Autodesk Fusion 360 part; units mm, degrees
(part 2 of 2)
sketch "Left" plane through (-18.285, 0, 0) normal (-1, 0, 0) x (0, 0, 1) in component "DXF Export"
  line L0 (-12.85, 17) -> (-12.85, 13)
  line L1 (-12.85, 13) -> (-17.35, 13)
  line L2 (-17.35, 13) -> (-17.35, 17)
  line L3 (-17.35, 17) -> (-12.85, 17)
  line L4 (23, -4) -> (23, 0)
  line L5 (23, 0) -> (27.5, 0)
  line L6 (27.5, 0) -> (27.5, 4.5)
  line L7 (27.5, 4.5) -> (31.5, 4.5)
  line L8 (31.5, 4.5) -> (31.5, 9)
  line L9 (31.5, 9) -> (27.5, 9)
  line L10 (27.5, 9) -> (27.5, 13.95)
  line L11 (27.5, 13.95) -> (26.8, 13.95)
  line L12 (26.8, 13.95) -> (26.8, 13.15)
  line L13 (26.8, 13.15) -> (25.4, 13.15)
  line L14 (25.4, 13.15) -> (25.4, 16.35)
  line L15 (25.4, 16.35) -> (26.8, 16.35)
  line L16 (26.8, 16.35) -> (26.8, 15.55)
  line L17 (26.8, 15.55) -> (27.5, 15.55)
  line L18 (27.5, 15.55) -> (27.5, 20.5)
  line L19 (27.5, 29.5) -> (23, 29.5)
  line L20 (23, 29.5) -> (23, 33.5)
  line L21 (23, 33.5) -> (18.5, 33.5)
  line L22 (18.5, 33.5) -> (18.5, 29.5)
  line L23 (18.5, 29.5) -> (0.8, 29.5)
  line L24 (0.8, 29.5) -> (0.8, 28.8)
  line L25 (0.8, 28.8) -> (1.6, 28.8)
  line L26 (1.6, 28.8) -> (1.6, 27.4)
  line L27 (1.6, 27.4) -> (-1.6, 27.4)
  line L28 (-1.6, 27.4) -> (-1.6, 28.8)
  line L29 (-1.6, 28.8) -> (-0.8, 28.8)
  line L30 (-0.8, 28.8) -> (-0.8, 29.5)
  line L31 (-0.8, 29.5) -> (-18.5, 29.5)
  line L32 (-18.5, 29.5) -> (-18.5, 33.5)
  line L33 (-18.5, 33.5) -> (-23, 33.5)
  line L34 (-23, 33.5) -> (-23, 29.5)
  line L35 (-23, 29.5) -> (-27.5, 29.5)
  line L36 (-27.5, 29.5) -> (-27.5, 25)
  line L37 (-27.5, 15.55) -> (-26.8, 15.55)
  line L38 (-26.8, 15.55) -> (-26.8, 16.35)
  line L39 (-26.8, 16.35) -> (-25.4, 16.35)
  line L40 (-25.4, 16.35) -> (-25.4, 13.15)
  line L41 (-25.4, 13.15) -> (-26.8, 13.15)
  line L42 (-26.8, 13.15) -> (-26.8, 13.95)
  line L43 (-26.8, 13.95) -> (-27.5, 13.95)
  line L44 (-27.5, 13.95) -> (-27.5, 9)
  line L45 (-27.5, 9) -> (-31.5, 9)
  line L46 (-31.5, 9) -> (-31.5, 4.5)
  line L47 (-31.5, 4.5) -> (-27.5, 4.5)
  line L48 (-27.5, 4.5) -> (-27.5, 0)
  line L49 (-27.5, 0) -> (-23, 0)
  line L50 (-23, 0) -> (-23, -4)
  line L51 (-23, -4) -> (-18.5, -4)
  line L52 (-18.5, -4) -> (-18.5, 0)
  line L53 (-18.5, 0) -> (-0.8, 0)
  line L54 (-0.8, 0) -> (-0.8, 0.7)
  line L55 (-0.8, 0.7) -> (-1.6, 0.7)
  line L56 (-1.6, 0.7) -> (-1.6, 2.1)
  line L57 (-1.6, 2.1) -> (1.6, 2.1)
  line L58 (1.6, 2.1) -> (1.6, 0.7)
  line L59 (1.6, 0.7) -> (0.8, 0.7)
  line L60 (0.8, 0.7) -> (0.8, 0)
  line L61 (0.8, 0) -> (18.5, 0)
  line L62 (18.5, 0) -> (18.5, -4)
  line L63 (18.5, -4) -> (23, -4)
  line L64 (27.5, 20.5) -> (31.5, 20.5)
  line L65 (31.5, 20.5) -> (31.5, 25)
  line L66 (31.5, 25) -> (27.5, 25)
  line L67 (27.5, 25) -> (27.5, 29.5)
  line L68 (-27.5, 25) -> (-31.5, 25)
  line L69 (-31.5, 25) -> (-31.5, 20.5)
  line L70 (-31.5, 20.5) -> (-27.5, 20.5)
  line L71 (-27.5, 20.5) -> (-27.5, 15.55)
sketch "Mid Plane" plane through (0, 17, 0) normal (0, 1, 0) x (-1, 0, 0) in component "DXF Export"
  line L0 (14.285, 27.5) -> (12.35, 27.5)
  line L1 (12.35, 27.5) -> (12.35, 31.5)
  line L2 (12.35, 31.5) -> (7.85, 31.5)
  line L3 (7.85, 31.5) -> (7.85, 27.5)
  line L4 (7.85, 27.5) -> (-14.285, 27.5)
  line L5 (-14.285, 27.5) -> (-14.285, 17.35)
  line L6 (-14.285, 17.35) -> (-18.285, 17.35)
  line L7 (-18.285, 17.35) -> (-18.285, 12.85)
  line L8 (-18.285, 12.85) -> (-14.285, 12.85)
  line L9 (-14.285, 12.85) -> (-14.285, -27.5)
  line L10 (-14.285, -27.5) -> (-12.35, -27.5)
  line L11 (-12.35, -27.5) -> (-12.35, -31.5)
  line L12 (-12.35, -31.5) -> (-7.85, -31.5)
  line L13 (-7.85, -31.5) -> (-7.85, -27.5)
  line L14 (-7.85, -27.5) -> (14.285, -27.5)
  line L15 (14.285, -27.5) -> (14.285, -17.35)
  line L16 (14.285, -17.35) -> (18.285, -17.35)
  line L17 (18.285, -17.35) -> (18.285, -12.85)
  line L18 (18.285, -12.85) -> (14.285, -12.85)
  line L19 (14.285, -12.85) -> (14.285, 27.5)
  line L20 (3.91, 10.1297) -> (-3.89, 10.1297)
  line L21 (-3.89, 10.1297) -> (-3.89, 24.1297)
  line L22 (-3.89, 24.1297) -> (3.91, 24.1297)
  line L23 (3.91, 24.1297) -> (3.91, 10.1297)
  line L24 (-10.165, 24.32) -> (-10.165, -24.52)
  line L25 (-10.165, -24.52) -> (-12.785, -24.52)
  line L26 (-12.785, -24.52) -> (-12.785, 24.32)
  line L27 (-12.785, 24.32) -> (-10.165, 24.32)
  line L28 (10.165, 24.32) -> (12.785, 24.32)
  line L29 (12.785, 24.32) -> (12.785, -24.52)
  line L30 (12.785, -24.52) -> (10.165, -24.52)
  line L31 (10.165, -24.52) -> (10.165, 24.32)
equation "d1 = object_length"
equation "d2 = object_width"
equation "d3 = tolerance_to_object"
equation "d4 = material_thickness + tolerance_to_object"
equation "d19 = object_height + tolerance_to_object * 2"
equation "d161 = 68.40 mm / 6"
equation "d199 = 4 mm"
equation "d210 = d199"
equation "d232 = d199"
equation "object_height = 26.5 mm"
equation "object_width = 25.57 mm"
equation "object_length = 52 mm"
equation "tolerance_to_object = 1.5 mm"
equation "pin_thickness = 4.5 mm"
equation "material_thickness = 4 mm"
equation "nut_width = 3.2 mm"
equation "nut_height = 1.4 mm"
equation "screw_length = 6.1 mm"
equation "screw_hole_diameter = 1.6 mm"
equation "d358 = object_height + 2 * tolerance_to_object"
equation "d361 = object_length / 2 + tolerance_to_object"
equation "d368 = d19 - pin_thickness"
equation "d385 = pin_thickness"
equation "d386 = pin_thickness"
equation "d387 = d386"
equation "d388 = pin_thickness"
equation "d389 = d388"
equation "d391 = pin_thickness"
equation "d392 = pin_thickness"
equation "d394 = d395"
equation "d395 = pin_thickness"
equation "d396 = d397"
equation "d397 = pin_thickness"
equation "d399 = pin_thickness"
equation "d401 = -d361"
equation "d402 = screw_hole_diameter"
equation "d403 = screw_hole_diameter"
equation "d404 = screw_hole_diameter"
equation "d405 = screw_hole_diameter"
equation "d406 = nut_width"
equation "d407 = nut_height"
equation "d409 = screw_hole_diameter"
equation "d410 = screw_hole_diameter"
equation "d411 = nut_width"
equation "d413 = nut_height"
equation "d420 = screw_length"
equation "d421 = material_thickness"
equation "d422 = material_thickness"
equation "d424 = screw_length"
equation "d425 = material_thickness"
equation "d426 = material_thickness"
equation "d427 = pin_thickness"
equation "d428 = pin_thickness"
equation "d429 = pin_thickness"
equation "d430 = pin_thickness"
equation "d433 = d428"
equation "d434 = d430"
equation "d435 = screw_hole_diameter"
equation "d436 = screw_hole_diameter"
equation "d437 = d399"
equation "d438 = d385"
equation "d439 = d391"
equation "d440 = d392"
equation "d441 = -material_thickness"
equation "d443 = material_thickness"
equation "d445 = material_thickness"
equation "d448 = -material_thickness"
equation "d450 = -object_width / 2 - tolerance_to_object"
equation "d451 = object_width / 2 + tolerance_to_object"
equation "d452 = nut_height"
equation "d453 = nut_width"
equation "d454 = screw_hole_diameter"
equation "d455 = screw_length"
equation "d456 = nut_width"
equation "d457 = screw_hole_diameter"
equation "d458 = nut_height"
equation "d459 = screw_length"
equation "d460 = screw_hole_diameter"
equation "d461 = nut_width"
equation "d462 = nut_height"
equation "d463 = screw_length"
equation "d464 = nut_height"
equation "d465 = screw_hole_diameter"
equation "d466 = nut_width"
equation "d467 = screw_length"
equation "d468 = material_thickness"
equation "d470 = -material_thickness"
equation "mid_layer_spacing = ( object_height + 2 * tolerance_to_object ) - 15 mm - tolerance_to_object"
equation "d473 = mid_layer_spacing"
equation "d474 = pin_thickness"
equation "d475 = pin_thickness"
equation "d476 = pin_thickness"
equation "d477 = pin_thickness"
equation "d478 = material_thickness"
equation "d480 = material_thickness"
equation "d482 = d427"
equation "d483 = d429"
equation "pin_rail_length = 48.84 mm"
equation "pin_rail_width = 2.62 mm"
equation "d489 = pin_rail_width"
equation "d490 = pin_rail_length"
equation "d491 = tolerance_to_object"
equation "d492 = pin_rail_width"
equation "d493 = pin_rail_length"
equation "d494 = tolerance_to_object"
equation "pin_rail_distance_to_back = 2.98 mm"
equation "d496 = pin_rail_distance_to_back"
equation "d497 = pin_rail_distance_to_back"
equation "jst_connector_width = 7.80 mm"
equation "jst_connector_length = 14.00 mm"
equation "d500 = jst_connector_width"
equation "d501 = jst_connector_length"
equation "d508 = 2 * tolerance_to_object"
equation "d509 = 2 * tolerance_to_object"
equation "d510 = tolerance_to_object"
equation "d513 = tolerance_to_object"
